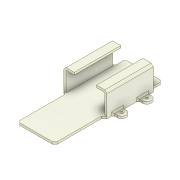
# Autodesk Inventor part: 3S lipo holder v2
Saved by Autodesk Inventor 2022 (Build 260153000, 153)
## iProperties
Created: 2024-07-16
Part Number: 3S lipo holder v2
Material: Generic
Document SubType Name: Modeling
Designer: david
Density: 1 g/cm^3
Appearance: Smooth - Ivory
Author: david
Autodesk Inventor part; units mm, degrees
ref_plane "YZ Plane" through (0, 0, 0) normal (1, 0, 0) x (0, 1, 0)
ref_plane "XZ Plane" through (0, 0, 0) normal (0, 1, 0) x (-1, 0, 0)
ref_plane "XY Plane" through (0, 0, 0) normal (0, 0, 1) x (1, 0, 0)
sketch "Sketch1" plane through (0, 0, 0) normal (0, 1, 0) x (-1, 0, 0)
  line L0 (-34.5, -17) -> (34.5, -17) construction
  line L1 (34.5, -17) -> (34.5, 17) construction
  line L2 (34.5, 17) -> (-34.5, 17) construction
  line L3 (-34.5, 17) -> (-34.5, -17) construction
  line L4 (-34.5, -17) -> (34.5, 17) construction
  line L5 (34.5, -17) -> (-34.5, 17) construction
  line L6 (-25, 27) -> (25, 27)
  line L7 (25, 27) -> (25, 23)
  line L8 (25, -27) -> (-25, -27)
  line L9 (-25, -27) -> (-25, -23)
  line L10 (-25, 27) -> (25, -27) construction
  line L11 (25, 27) -> (-25, -27) construction
  line L12 (-34.5, 17) -> (34.5, 17) construction
  line L13 (-34.5, 11) -> (-25, 11)
  line L14 (34.5, 23) -> (25, 23)
  arc A0 (-34.5, 23) -> (-34.5, 11) centre (-34.5, 17) ccw
  arc A1 (34.5, 11) -> (34.5, 23) centre (34.5, 17) ccw
  line L15 (56.7, 0) -> (-56.7, 0) projected
  line L16 (34.5, -17) -> (-34.5, -17) construction
  line L17 (-34.5, -17) -> (34.5, -17) construction
  line L18 (-34.5, -11) -> (-25, -11)
  line L19 (34.5, -23) -> (25, -23)
  arc A2 (-34.5, -11) -> (-34.5, -23) centre (-34.5, -17) ccw
  arc A3 (34.5, -23) -> (34.5, -11) centre (34.5, -17) ccw
  line L20 (25, 23) -> (25, 17)
  line L21 (25, 11) -> (34.5, 11)
  line L22 (25, -11) -> (34.5, -11)
  line L23 (25, -23) -> (25, -27)
  line L24 (-25, -23) -> (-25, -11)
  line L25 (-25, -11) -> (-25, 11)
  line L26 (-25, 23) -> (-25, 27)
  line L27 (25, 17) -> (25, -11)
  line L28 (25, 23) -> (-25, 23) construction
  line L29 (-25, 23) -> (-34.5, 23)
  line L30 (-25, 11) -> (-25, 23)
  line L31 (-25, -23) -> (-34.5, -23)
  line L32 (-25, -11) -> (25, -11) construction
  line L33 (25, -23) -> (-25, -23) construction
  line L34 (-25, 11) -> (25, 11) construction
  line L35 (25, -11) -> (25, -23)
  line L36 (-29, -31.32) -> (29, -31.32)
  line L37 (29, -31.32) -> (29, 31.32)
  line L38 (29, 31.32) -> (-29, 31.32)
  line L39 (-29, 31.32) -> (-29, -31.32)
  line L40 (-29, -31.32) -> (29, 31.32) construction
  line L41 (29, -31.32) -> (-29, 31.32) construction
  line L42 (-25, -27) -> (25, -27)
  line L43 (25, -27) -> (25, 97.68)
  line L44 (25, 97.68) -> (-25, 97.68)
  line L45 (-25, 97.68) -> (-25, -27)
  line L46 (25, -27) -> (-25, -27)
  line L47 (-25, -27) -> (-25, -47.32)
  line L48 (-25, -47.32) -> (25, -47.32)
  line L49 (25, -47.32) -> (25, -27)
  point P0 (0, 0)
  point P1 (-34.5, 17)
  point P2 (0, 17)
  point P3 (-34.5, -17)
  point P4 (0, -17)
  point P5 (29, -11)
  point P6 (29, 11)
  point P7 (-29, 11)
  point P8 (-29, -11)
  point P9 (29, 23)
  point P10 (-29, 23)
  point P11 (-29, -23)
  point P12 (29, -23)
  point P13 (-25, 31.32)
  point P14 (25, 31.32)
  point P15 (25, -31.32)
  point P16 (-25, -31.32)
  dimension "d0" = 34
  dimension "d1" = 69
  dimension "d2" = 50
  dimension "d3" = 10
  dimension "d4" = 6
  dimension "d41" = 145
  dimension "d42" = 16
  dimension "d43" = 4
  constraints: 102 end point, 43 parallel, 12 tangent, 8 midpoint, 8 perpendicular, 8 point on circle, 8 symmetric about line, 6 collinear, 6 horizontal, 6 point on line, 4 centre point, 2 coincident
  measures "d0" distance of L0.end L1.end
  measures "d1" distance of L1.end L2.end
  measures "d2" distance of L8.start L8.end
  measures "d3" distance between parallel lines of L2 L6
  measures "d4" radius of A1
  measures "d41" distance between parallel lines of L48 L44
  measures "d42" distance between parallel lines of L48 L36
  measures "d43" distance between parallel lines of L37 L43
extrude "Extrusion1" add sketch "Sketch1" along normal blind 3
sketch "Sketch2" plane through (0, 3, 0) normal (0, 1, 0) x (1, 0, 0)
  arc A0 (-34.5, -11) -> (-34.5, -23) centre (-34.5, -17) ccw projected
  arc A1 (-34.5, 23) -> (-34.5, 11) centre (-34.5, 17) ccw projected
  arc A2 (34.5, 11) -> (34.5, 23) centre (34.5, 17) ccw projected
  arc A3 (34.5, -23) -> (34.5, -11) centre (34.5, -17) ccw projected
  point P0 (0, 0)
  constraints: 4 coincident
hole "Hole1" at (-34.5, 3, 17) at (-34.5, 3, -17) at (34.5, 3, -17) at (34.5, 3, 17) direction (0, -1, 0) diameter 3.4 depth 6
sketch "Sketch5" plane through (29, 0, -31.32) normal (0, 0, -1) x (-1, 0, 0)
  line L0 (0, 0) -> (0, 3) projected
  line L1 (0, 3) -> (4, 3) projected
  line L2 (58, 3) -> (58, 0) projected
  line L3 (58, 0) -> (54, 0) projected
  line L4 (0, 3) -> (58, 3) projected
  line L5 (58, 3) -> (58, 32.5)
  line L6 (58, 32.5) -> (44, 32.5)
  line L7 (44, 32.5) -> (44, 28.5)
  line L8 (44, 28.5) -> (54, 28.5)
  line L9 (54, 28.5) -> (54, 0)
  line L10 (29, -6.6) -> (29, 39.6) projected
  line L11 (0, 3) -> (0, 0)
  line L12 (0, 3) -> (0, 32.5)
  line L13 (0, 32.5) -> (14, 32.5)
  line L14 (14, 32.5) -> (14, 28.5)
  line L15 (14, 28.5) -> (4, 28.5)
  line L16 (4, 28.5) -> (4, 0)
  line L17 (0, 0) -> (58, 0) projected
  line L18 (4, 0) -> (4, 3) projected
  line L19 (54, 0) -> (4, 0) projected
  line L20 (54, 3) -> (54, 0) projected
  line L21 (54, 3) -> (58, 3) projected
  line L22 (4, 0) -> (0, 0) projected
  line L23 (4, 3) -> (54, 3) projected
  line L24 (4, 0) -> (4, 3) projected
  line L25 (4, 3) -> (4, 0)
  line L26 (4, 0) -> (0, 0)
  point P0 (29, 0)
  point P1 (3.7037, 0)
  point P2 (53.4074, 3)
  point P3 (4, 0)
  point P4 (4, 3)
  point P5 (54, 3)
  dimension "d21" = 4
  dimension "d22" = 25.5
  dimension "d23" = 10
  constraints: 26 end point, 5 symmetric about line, 4 perpendicular, 2 collinear, 1 vertical, 1 other
  measures "d21" distance of L6.end L7.end
  measures "d22" distance between parallel lines of L1 L8
  measures "d23" distance between parallel lines of L9 L7
extrude "Extrusion2" add sketch "Sketch5" against normal up to surface (62.64 mm away) contours L0 L1 L16 L17 | L12 L13 L14 L15 L16 L1 | L9 L8 L7 L6 L5 L4
chamfer "Chamfer2" distance 2 angle 45 12 edges at (-29, 3, -17) (-29, 3, 17) (29, 3, 17) (29, 3, -17) (29, 1.5, 23) (29, 1.5, -23) (29, 1.5, -11) (29, 1.5, 11) (-29, 1.5, -11) (-29, 1.5, 23) (-29, 1.5, 11) (-29, 1.5, -23)
chamfer "Chamfer3" distance 3 angle 45 2 edges at (29, 32.5, 0) (-29, 32.5, 0)
chamfer "Chamfer4" distance 3.7037 angle 45 4 edges at (25, 1.5, 31.32) (-25, 1.5, 31.32) (25, 1.5, -31.32) (-25, 1.5, -31.32)
chamfer "Chamfer5" distance 3 angle 45 4 edges at (25, 1.5, 97.68) (-25, 1.5, 97.68) (25, 1.5, -47.32) (-25, 1.5, -47.32)
thicken "Thicken3" operation add thickness 1 both sides no extend neighbours yes toward (0, 1, 0) faces at (21.6667, 28.5, 10.44) (25, 11.5, 10.44)
thicken "Thicken4" operation add thickness 1 both sides no extend neighbours yes toward (0, 1, 0) faces at (-18.3333, 28.5, 10.44) (-25, 20, 10.44)
equation "\"d21\" = d20"
equation "\"d50\" = d48"
equation "\"d51\" = d48"
equation "\"d20\" = d14"
equation "\"d48\" = 1"
equation "\"d14\" = 4"
body "Solid1"
